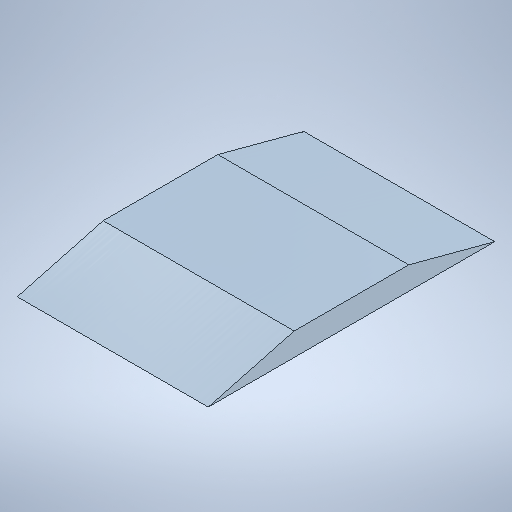
# Autodesk Inventor part: ramp
Saved by Autodesk Inventor 2025.3 (Build 293356030, 356C)
## iProperties
Created: 2026-07-06
Part Number: ramp
Material: Brass
Document SubType Name: Modeling
Designer: user
Density: 8.49 g/cm^3
Appearance: Steel Blue
Author: user
Autodesk Inventor part; units mm, degrees
ref_plane "YZ Plane" through (0, 0, 0) normal (1, 0, 0) x (0, 1, 0)
ref_plane "XZ Plane" through (0, 0, 0) normal (0, 1, 0) x (-1, 0, 0)
ref_plane "XY Plane" through (0, 0, 0) normal (0, 0, 1) x (1, 0, 0)
sketch "Sketch1" plane through (0, 0, 0) normal (1, 0, 0) x (0, 1, 0)
  line L0 (0, 0) -> (0, -225)
  line L1 (0, -225) -> (60, -225)
  line L2 (60, -225) -> (0, 0)
  line L3 (60, -225) -> (60, -525)
  line L4 (60, -525) -> (0, -750)
  line L5 (0, -750) -> (0, -225)
  line L6 (60, -525) -> (0, -525)
  dimension "d0" = 225
  dimension "d1" = 60
  dimension "d2" = 300
  dimension "d3" = 225
  constraints: 14 end point, 3 vertical, 1 horizontal, 1 perpendicular, 1 point on line
  measures "d0" distance of L0.start L0.end
  measures "d1" distance of L0.end L1.end
  measures "d2" distance of L1.end L3.end
  measures "d3" distance of L6.end L4.end
extrude "Extrusion1" add sketch "Sketch1" along normal blind 500
body "Solid1"
